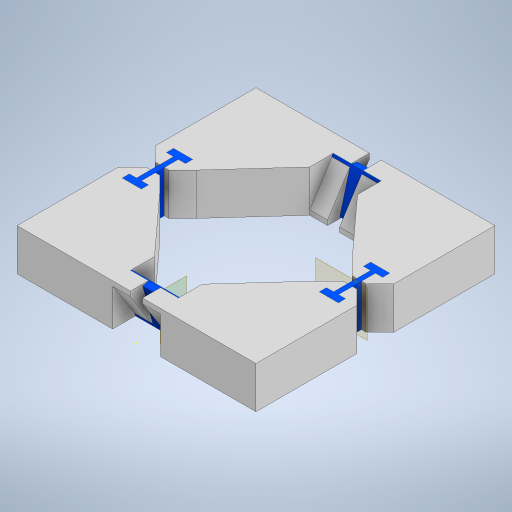
# Autodesk Inventor part: Modular_Bending_v3
Saved by Autodesk Inventor 2023 (Build 270158000, 158)
## iProperties
Created: 2022-07-18
Part Number: Modular_Bending_v3
Material: Generic
Document SubType Name: Modeling
Designer: hci-u
Density: 1 g/cm^3
Appearance: Default
Author: hci-u
Autodesk Inventor part; units mm, degrees
ref_plane "YZ Plane" through (0, 0, 0) normal (1, 0, 0) x (0, 1, 0)
ref_plane "XZ Plane" through (0, 0, 0) normal (0, 1, 0) x (-1, 0, 0)
sketch "Sketch1" plane through (0, 0, 0) normal (0, 1, 0) x (-1, 0, 0)
  line L0 (0, 0) -> (7, 0)
  line L1 (7, 0) -> (7, -7) construction
  line L2 (7, -7) -> (0, -7) construction
  line L3 (0, -7) -> (0, 0)
  line L4 (7, 0) -> (16, 0)
  line L5 (16, -7) -> (7, -7)
  line L6 (7, -7) -> (7, -16.9)
  line L7 (7, -16.9) -> (3.9, -20)
  line L8 (3.9, -20) -> (3.9, -16.9)
  line L9 (3.1, -16.9) -> (3.1, -20)
  line L10 (3.1, -20) -> (0, -16.9)
  line L11 (0, -16.9) -> (0, -7)
  line L12 (3.9, -20) -> (3.1, -20)
  line L13 (3.5, -15.7) -> (3.5, -20) construction
  line L14 (7, -16.9) -> (3.9, -16.9) construction
  line L15 (3.1, -16.9) -> (0, -16.9) construction
  line L16 (3.1, 0) -> (3.1, -20) construction
  line L17 (4.65, -19.25) -> (3.9, -19.25)
  line L18 (3.1, -19.25) -> (2.35, -19.25)
  line L19 (3.9, -20) -> (4.275, -19.25) construction
  line L20 (16, -7) -> (16, 0)
  line L21 (0, -3.5) -> (20, -3.5) construction
  line L22 (7, -16.9) -> (16, -7)
  line L23 (5.1, -15.7) -> (1.9, -15.7)
  line L24 (1.9, -15.7) -> (1.9, -16.9)
  line L25 (5.1, -16.9) -> (5.1, -15.7)
  line L26 (1.9, -16.9) -> (3.1, -16.9)
  line L27 (3.9, -16.9) -> (5.1, -16.9)
  point P0 (3.5, -7)
  dimension "L_2" = 20
  dimension "wLink" = 7
  dimension "wFlex" = 0.8
  dimension "LenFlex" = 0.75
  dimension "LenDiagTPU" = 4
  dimension "d66" = 45
  dimension "d101" = 1.2
  constraints: 56 end point, 13 point on line, 9 perpendicular, 6 parallel, 5 horizontal, 5 midpoint, 3 collinear, 1 coincident, 1 vertical, 2 other
  measures "L_2" distance between parallel lines of L0 L12
  measures "wLink" distance between parallel lines of L11 L6
  measures "wFlex" distance between parallel lines of L16 L8
  measures "LenFlex" distance from line of L7.end L17
  measures "LenDiagTPU" distance from line of L20 L21.end
  measures "d66" angle of L8 L7
  measures "d101" distance of L23.end L24.end
extrude "Extrusion1" add sketch "Sketch1" along normal blind 7 contours L0 L4 L20 L5 L6 L7 L17 L8 L27 L25 L23 L24 L26 L9 L18 L10 L11 L3 | L22 L6 L5
ref_plane "Work Plane5" through (-20, 0, -7) normal (-1, 0, 0) x (0, 0, 1)
sketch "Sketch10" plane through (-16, 0, -7) normal (-1, 0, 0) x (0, 0, 1)
  line L0 (2.2078, 0.2228) -> (4.0195, 6.9843) construction
  line L1 (4.0195, 6.9843) -> (4.7922, 6.7772) construction
  line L2 (4.7922, 6.7772) -> (2.9805, 0.0157) construction
  line L3 (2.9805, 0.0157) -> (2.2078, 0.2228) construction
  line L4 (2.5941, 0.1193) -> (4.4059, 6.8807) construction
  line L5 (7, 0) -> (7, 7) projected
  line L6 (7, 3.5) -> (3.5, 3.5) construction
  line L7 (0, 0) -> (7, 0) projected
  line L8 (3.5, 0) -> (3.5, 3.5) construction
  line L9 (0, 7) -> (7, 7) projected
  line L10 (3.9608, 7) -> (4.0195, 6.9843) construction
  line L11 (4.7922, 6.7772) -> (7, 6.1856) construction
  line L12 (2.2078, 0.2228) -> (0, 0.8144) construction
  line L13 (0, 0) -> (0, 7) projected
  line L14 (2.9805, 0.0157) -> (3.0392, 0) construction
  line L15 (3.0392, 0) -> (7, 6.1856)
  line L16 (0, 0.8144) -> (3.9608, 7)
  line L17 (0, 0.8144) -> (0, 0)
  line L18 (-9.9, 0) -> (0, 0) projected
  line L19 (3.0392, 0) -> (0, 0)
  line L20 (3.9608, 7) -> (7, 7)
  line L21 (7, 6.1856) -> (7, 7)
  dimension "d102" = 0.8
  dimension "d103" = 75
  constraints: 34 end point, 6 collinear, 6 point on line, 5 midpoint, 3 perpendicular, 2 horizontal, 1 equal length, 1 parallel, 1 vertical
  measures "d102" distance between parallel lines of L2 L0
  measures "d103" angle of L4 L6
extrude "Extrusion9" add sketch "Sketch10" along normal blind 3 contours L15 L7 L13 L16 L9 L5
sketch "Sketch11" plane through (-20, 0, -7) normal (-1, 0, 0) x (0, 0, 1)
  line L0 (2.0146, 0.2746) -> (3.8263, 7.036)
  line L1 (3.8263, 7.036) -> (4.9854, 6.7254)
  line L2 (4.9854, 6.7254) -> (3.1737, -0.036)
  line L3 (3.1737, -0.036) -> (2.0146, 0.2746)
  line L4 (3.8263, 7.036) -> (3.9608, 7)
  line L5 (3.1737, -0.036) -> (3.0392, 0)
  point P0 (0, 0.8144)
  dimension "d104" = 1.2
  constraints: 12 end point, 3 perpendicular, 3 point on line, 2 parallel
  measures "d104" distance between parallel lines of L2 L0
extrude "Extrusion10" cut sketch "Sketch11" against normal blind 4
sketch "Sketch22" plane through (0, 7, 0) normal (0, 1, 0) x (1, 0, 0)
  line L0 (-5.1, 15.7) -> (-5.1, 16.9) projected
  line L1 (-1.9, 15.7) -> (-5.1, 15.7) projected
  line L2 (-5.1, 15.7) -> (-1.9, 15.7)
  line L3 (-1.9, 16.9) -> (-1.9, 15.7) projected
  line L4 (-1.9, 15.7) -> (-1.9, 16.9)
  line L5 (-1.9, 16.9) -> (-3.1, 16.9)
  line L6 (-3.1, 16.9) -> (-3.1, 20)
  line L7 (-3.1, 20) -> (-3.9, 20)
  line L8 (-3.9, 16.9) -> (-3.9, 19.25) projected
  line L9 (-3.9, 20) -> (-3.9, 16.9)
  line L10 (-3.9, 16.9) -> (-5.1, 16.9)
  line L11 (-5.1, 16.9) -> (-5.1, 15.7)
  line L12 (4, 20) -> (-24, 20) projected
  point P0 (0, 0)
  constraints: 16 end point, 4 perpendicular, 2 collinear, 2 point on line, 1 horizontal
extrude "Extrusion19" add sketch "Sketch22" against normal up to surface (7 mm away) separate body
sketch "Sketch23" plane through (-16, 0, 0) normal (-1, 0, 0) x (0, 0, 1)
  line L0 (-2.0146, 6.7254) -> (-3.7129, 0.3871) projected
  line L1 (-2.0146, 6.7254) -> (-3.1737, 7.036)
  line L2 (-4.9854, 0.2746) -> (-3.2871, 6.6129) projected
  line L3 (-3.1737, 7.036) -> (-4.9854, 0.2746)
  line L4 (-4.9854, 0.2746) -> (-3.8263, -0.036)
  line L5 (-3.8263, -0.036) -> (-2.0146, 6.7254)
  point P0 (0, 0)
  point P1 (-3.7129, 0.3871)
  constraints: 8 end point, 3 perpendicular, 1 collinear
extrude "Extrusion20" add sketch "Sketch23" along normal up to surface (4 mm away) bodies 2
sketch "Sketch25" plane through (-20, 0.2746, -4.9854) normal (-1, 0, 0) x (0, -0.2588, 0.9659)
  point P0 (4.8866, 1.0251)
sketch "Sketch26" plane through (-20, 0.2746, -4.9854) normal (-1, 0, 0) x (0, -0.2588, 0.9659)
  line L0 (3.0749, 7.7866) -> (-13.2493, 3.4126) projected
  line L1 (3.0749, 7.7866) -> (4.8866, 1.0251)
  line L2 (4.8866, 1.0251) -> (-1.8749, -0.7866)
  line L3 (-2.0856, 0) -> (-3.6866, 5.9749) projected
  line L4 (-1.8749, -0.7866) -> (-3.6866, 5.9749)
  line L5 (-3.6866, 5.9749) -> (3.0749, 7.7866)
  line L6 (-4.299, 6.3284) -> (-2.2284, -1.399)
  line L7 (-2.2284, -1.399) -> (5.499, 0.6716)
  line L8 (5.499, 0.6716) -> (3.4284, 8.399)
  line L9 (3.4284, 8.399) -> (-4.299, 6.3284)
  line L10 (-0.3059, 6.8807) -> (-0.4353, 7.3637) construction
  line L11 (4.8866, 1.0251) -> (3.0749, 7.7866) projected
  line L12 (3.9807, 4.4059) -> (4.4637, 4.5353) construction
  point P0 (-2.0856, 0)
  dimension "d109" = 0.5
  constraints: 20 end point, 9 perpendicular, 4 midpoint, 1 collinear, 1 parallel
  measures "d109" distance between parallel lines of L1 L8
extrude "Extrusion21" cut sketch "Sketch26" against normal up to surface (4 mm away) bodies 2
mirror "Mirror1" about plane through (-20, 0, -7) normal (-1, 0, 0) of "Extrusion1", "Extrusion9", "Extrusion10" bodies 1
sketch "Sketch15" plane through (0, 7, 0) normal (0, 1, 0) x (1, 0, 0)
  line L0 (0.1, 17) -> (-2.9, 20) construction
  line L1 (0, 16.9) -> (-2.35, 19.25) projected
  line L2 (-3.1, 19.25) -> (-3.1, 16.9) construction
  line L3 (-2.9, 20) -> (-2.9, 17.1) construction
  point P0 (-2.35, 19.25)
  point P1 (-2.9, 18.4748)
  constraints: 2 end point, 1 vertical, 5 other
ref_plane "Work Plane10" through (-16, 0, -20) normal (0, 0, 1) x (1, 0, 0)
mirror "Mirror2" about plane through (-16, 0, -20) normal (0, 0, 1) of "Extrusion1", "Mirror1", "Extrusion9", "Extrusion10" bodies 1
mirror "Mirror10" about plane through (-1.8, 7, -20) normal (0, 0, -1) of "Extrusion19", "Extrusion20", "Extrusion21" bodies 2
mirror "Mirror11" about plane through (-20, 0, -7) normal (-1, 0, 0) of "Extrusion19", "Extrusion20", "Mirror10", "Extrusion21" bodies 2
ref_plane "Work Plane7" through (-1.8, 7, -20) normal (0, 0, -1) x (-1, 0, 0)
body "Solid1"
body "Solid2"
